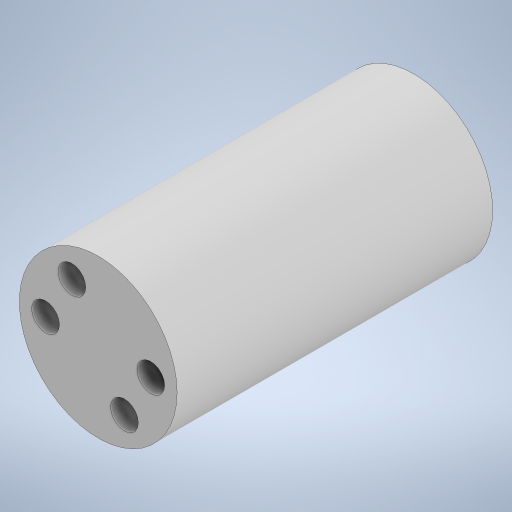
# Autodesk Inventor part: Crankshaft
Saved by Autodesk Inventor 2023 (Build 270158000, 158)
## iProperties
Created: 2022-10-29
Part Number: Crankshaft
Material: Generic
Document SubType Name: Modeling
Designer: tommy
Density: 1 g/cm^3
Appearance: Default
Author: tommy
Autodesk Inventor part; units mm, degrees
ref_plane "YZ Plane" through (0, 0, 0) normal (1, 0, 0) x (0, 1, 0)
ref_plane "XZ Plane" through (0, 0, 0) normal (0, 1, 0) x (-1, 0, 0)
ref_plane "XY Plane" through (0, 0, 0) normal (0, 0, 1) x (1, 0, 0)
sketch "Sketch1" plane through (0, 0, 0) normal (0, 0, 1) x (1, 0, 0)
  circle A0 centre (3.175, -5.4993) radius 1.6764
  circle A1 centre (-3.175, 5.4993) radius 1.6764
  circle A2 centre (0, 0) radius 9.525
  circle A3 centre (-6.35, 0) radius 1.6764
  circle A4 centre (6.35, 0) radius 1.6764
  circle A5 centre (-6.35, 0) radius 1.6764
  circle A6 centre (6.35, 0) radius 1.6764
  point P0 (-9.525, 0)
  point P1 (9.525, 0)
  dimension "d69" = 3.3528
  dimension "d70" = 3.3528
  dimension "d75" = 3.3528
  dimension "d76" = 3.3528
  dimension "d77" = 3.3528
  dimension "d78" = 3.3528
  constraints: 6 centre point, 1 horizontal alignment, 2 other
  measures "d69" diameter of A1
  measures "d70" diameter of A0
  measures "d75" diameter of A4
  measures "d76" diameter of A3
  measures "d77" diameter of A6
  measures "d78" diameter of A5
extrude "Extrusion14" add sketch "Sketch1" along normal blind 38.1
body "Solid5"
